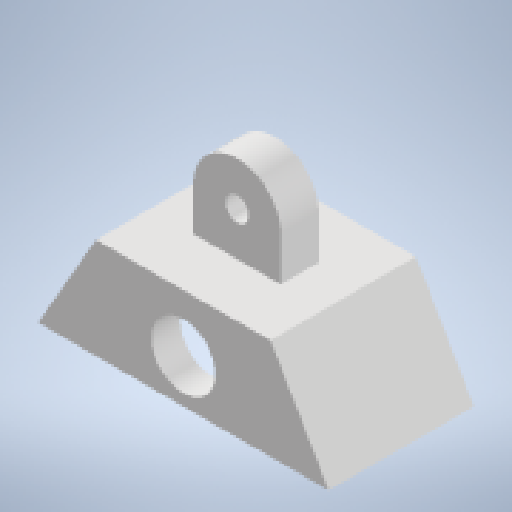
# Autodesk Inventor part: center_wheel_well
Saved by Autodesk Inventor 2024 (Build 280153000, 153)
## iProperties
Created: 2025-11-24
Part Number: center_wheel_well
Material: Generic
Document SubType Name: Modeling
Designer: Aidan
Density: 1 g/cm^3
Appearance: Default
Author: Aidan
Autodesk Inventor part; units mm, degrees
ref_plane "YZ Plane" through (0, 0, 0) normal (1, 0, 0) x (0, 1, 0)
ref_plane "XZ Plane" through (0, 0, 0) normal (0, 1, 0) x (-1, 0, 0)
ref_plane "XY Plane" through (0, 0, 0) normal (0, 0, 1) x (1, 0, 0)
sketch "Sketch1" plane through (0, 0, 0) normal (0, 0, 1) x (1, 0, 0)
  line L0 (0, 0) -> (20, 34.641)
  line L1 (20, 34.641) -> (80, 34.641)
  line L2 (80, 34.641) -> (100, 0)
  line L3 (100, 0) -> (0, 0)
  dimension "d2" = 40
  dimension "d3" = 60
  dimension "d4" = 40
  dimension "d5" = 100
  constraints: 8 end point, 1 horizontal, 1 parallel
  measures "d2" distance of L0.start L0.end
  measures "d3" distance of L0.end L1.end
  measures "d4" distance of L1.end L2.end
  measures "d5" distance of L2.end L0.start
extrude "Extrusion1" add sketch "Sketch1" along normal blind 50
sketch "Sketch2" plane through (20, 34.641, 0) normal (0, 1, 0) x (1, 0, 0)
  line L0 (45, -10) -> (15, -10)
  line L1 (15, -10) -> (15, -40)
  line L2 (15, -40) -> (45, -40)
  line L3 (45, -40) -> (45, -10)
  line L4 (60, 0) -> (0, 0) projected
  line L5 (-20, 0) -> (-20, -50) projected
  line L6 (45, -20) -> (15, -20)
  line L7 (45, -30) -> (15, -30)
  point P0 (30, 0)
  point P1 (45, -25)
  point P2 (30, -40)
  dimension "d8" = 30
  dimension "d9" = 30
  dimension "d10" = 25
  dimension "d11" = 50
  dimension "d31" = 10
  dimension "d32" = 10
  constraints: 12 end point, 4 point on line, 3 midpoint, 3 perpendicular, 2 parallel, 1 horizontal
  measures "d8" distance of L2.end L1.end
  measures "d9" distance of L1.end L0.end
  measures "d10" vertical distance of point (30, 0) point (45, -25)
  measures "d11" distance from line of L5 point (30, -40)
  measures "d31" distance between parallel lines of L0 L6
  measures "d32" distance between parallel lines of L2 L7
extrude "Extrusion2" add sketch "Sketch2" along normal blind 30 contours L3 L6 L1 L0 | L3 L2 L1 L7
sketch "Sketch3" plane through (0, 0, 0) normal (0, -1, 0) x (1, 0, 0)
  line L0 (22.5, 10) -> (77.5, 10)
  line L1 (77.5, 10) -> (77.5, 40)
  line L2 (77.5, 40) -> (22.5, 40)
  line L3 (22.5, 40) -> (22.5, 10)
  line L4 (0, 0) -> (0, 50) projected
  line L5 (0, 50) -> (100, 50) projected
  point P0 (50, 10)
  point P1 (22.5, 25)
  dimension "d14" = 55
  dimension "d15" = 30
  dimension "d16" = 50
  dimension "d17" = 25
  constraints: 8 end point, 2 midpoint, 2 parallel, 1 horizontal, 1 perpendicular
  measures "d14" distance of L2.end L1.end
  measures "d15" distance of L1.end L0.end
  measures "d16" distance from line of L4 point (50, 10)
  measures "d17" distance from line of L5 point (22.5, 25)
extrude "Extrusion3" cut sketch "Sketch3" against normal blind 30
sketch "Sketch4" plane through (0, 0, 50) normal (0, 0, 1) x (1, 0, 0)
  circle A0 centre (50, 10) radius 4.05
  line L0 (0, 0) -> (100, 0) projected
  dimension "d20" = 8.1
  dimension "d21" = 10
  dimension "d22" = 50
  constraints: 1 centre point
  measures "d20" diameter of A0
  measures "d21" distance from line of L0 A0.centre
  measures "d22" horizontal distance of L0.start A0.centre
extrude "Extrusion4" cut sketch "Sketch4" against normal up to surface (50 mm away)
sketch "Sketch5" plane through (35, 34.641, 40) normal (0, 0, 1) x (1, 0, 0)
  circle A0 centre (15, 15) radius 4.05
  line L0 (30, 0) -> (30, 30) projected
  line L1 (0, 30) -> (30, 30) projected
  line L2 (0, 0) -> (0, 30) projected
  arc A1 (30, 15) -> (0, 15) centre (15, 15) ccw
  line L3 (0, 15) -> (0, 30)
  line L4 (30, 30) -> (30, 15)
  line L5 (30, 30) -> (0, 30)
  point P0 (-35, -34.641)
  point P1 (15, 30)
  dimension "d25" = 8.1
  dimension "d26" = 15
  dimension "d27" = 15
  dimension "d28" = 15
  constraints: 6 end point, 2 centre point, 2 collinear, 2 midpoint, 2 point on circle
  measures "d25" diameter of A0
  measures "d26" distance from line of L0 A0.centre
  measures "d27" distance from line of L1 A0.centre
  measures "d28" radius of A1
extrude "Extrusion5" cut sketch "Sketch5" against normal up to surface (30 mm away)
sketch "Sketch6" plane through (0, 30, 0) normal (0, -1, 0) x (1, 0, 0)
  line L0 (77.5, 40) -> (77.5, 10) projected
  line L1 (22.5, 40) -> (77.5, 40) projected
  line L2 (22.5, 10) -> (22.5, 40) projected
  line L3 (77.5, 10) -> (22.5, 10) projected
  line L4 (77.5, 20) -> (22.5, 20)
  line L5 (22.5, 20) -> (22.5, 30)
  line L6 (22.5, 30) -> (77.5, 30)
  line L7 (77.5, 30) -> (77.5, 20)
  point P0 (0, 0)
  point P1 (22.5, 20)
  dimension "d33" = 10
  dimension "d34" = 10
  constraints: 8 end point, 2 parallel, 1 collinear, 1 horizontal, 1 perpendicular, 1 point on line
  measures "d33" distance between parallel lines of L3 L4
  measures "d34" distance between parallel lines of L1 L6
extrude "Extrusion6" cut sketch "Sketch6" against normal up to surface (4.641 mm away) contours L0 L4 L2 L6
body "Solid1"
